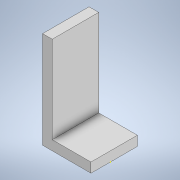
# Autodesk Inventor part: Part9
Saved by Autodesk Inventor 2021 (Build 250183000, 183)
## iProperties
Created: 2021-07-04
Part Number: Part9
Material: Generic
Document SubType Name: Modeling
Designer: VK
Density: 1 g/cm^3
Appearance: Default
Author: VK
Autodesk Inventor part; units mm, degrees
ref_plane "YZ Plane" through (0, 0, 0) normal (1, 0, 0) x (0, 1, 0)
ref_plane "XZ Plane" through (0, 0, 0) normal (0, 1, 0) x (-1, 0, 0)
ref_plane "XY Plane" through (0, 0, 0) normal (0, 0, 1) x (1, 0, 0)
sketch "Sketch1" plane through (0, 0, 0) normal (0, 1, 0) x (-1, 0, 0)
  line L0 (0, 0) -> (25, 0)
  line L1 (25, 0) -> (25, -10)
  line L2 (25, -10) -> (0, -10)
  line L3 (0, -10) -> (0, 0)
  dimension "d0" = 25
  dimension "d1" = 10
  constraints: 8 end point, 2 parallel, 1 horizontal, 1 perpendicular
  measures "d0" distance of L1.end L2.end
  measures "d1" distance of L0.end L1.end
extrude "Extrusion1" add sketch "Sketch1" along normal blind 5
sketch "Sketch2" plane through (0, 5, 0) normal (0, 1, 0) x (1, 0, 0)
  line L0 (-25, 10) -> (-25, 0) projected
  line L1 (-25, 0) -> (0, 0) projected
  line L2 (-25, 10) -> (-20, 10)
  line L3 (-20, 10) -> (-20, 0)
  line L4 (-20, 0) -> (-25, 0)
  line L5 (-25, 0) -> (-25, 10)
  dimension "d4" = 5
  constraints: 8 end point, 2 parallel, 1 horizontal, 1 perpendicular, 1 point on line
  measures "d4" distance of L3.end L4.end
extrude "Extrusion2" add sketch "Sketch2" along normal blind 45
sketch "Sketch3" plane through (0, 0, -10) normal (0, 0, -1) x (-1, 0, 0)
  point P0 (0, 0)
sketch "Sketch4" plane through (0, 0, -10) normal (0, 0, -1) x (-1, 0, 0)
  line L0 (0, 5) -> (20, 5) projected
  line L1 (0, 0) -> (0, 5) projected
  line L2 (0, 5) -> (0, 0)
  line L3 (0, 0) -> (25, 0)
  line L4 (25, 0) -> (25, 50) projected
  line L5 (25, 0) -> (25, 50)
  line L6 (20, 50) -> (25, 50) projected
  line L7 (25, 50) -> (20, 50)
  line L8 (20, 5) -> (20, 50) projected
  line L9 (20, 50) -> (20, 5)
  line L10 (20, 5) -> (0, 5)
  constraints: 12 end point, 3 perpendicular, 2 collinear, 1 vertical
extrude "Extrusion3" add sketch "Sketch4" along normal blind 14
body "Solid1"
